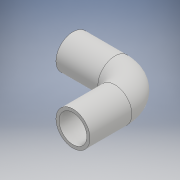
# Autodesk Inventor part: Effector Wire Conduit
Saved by Autodesk Inventor 2018 (Build 220112000, 112)
## iProperties
Created: 2018-05-02
Part Number: Effector Wire Conduit
Material: Generic
Document SubType Name: Modeling
Designer: elect
Density: 1 g/cm^3
Appearance: Default
Author: elect
Autodesk Inventor part; units mm, degrees
ref_plane "YZ Plane" through (0, 0, 0) normal (1, 0, 0) x (0, 1, 0)
ref_plane "XZ Plane" through (0, 0, 0) normal (0, 1, 0) x (-1, 0, 0)
ref_plane "XY Plane" through (0, 0, 0) normal (0, 0, 1) x (1, 0, 0)
sketch "Sketch1" plane through (0, 0, 0) normal (0, 1, 0) x (-1, 0, 0)
  circle A0 centre (0, 0) radius 8.125
  circle A1 centre (0, 0) radius 6.625
  dimension "d0" = 16.25
  dimension "d1" = 13.25
  constraints: 2 centre point, 2 coincident
  measures "d0" diameter of A0
  measures "d1" diameter of A1
sketch "Sketch3" plane through (0, 0, 0) normal (0, 0, 1) x (1, 0, 0)
  line L0 (8.125, 0) -> (8.125, 20)
  line L1 (8.125, 0) -> (28.125, 0) construction
  arc A0 (8.125, 20) -> (-11.875, 40) centre (-11.875, 20) ccw
  line L2 (-11.875, 40) -> (-31.875, 40)
  point P0 (0, 0)
  dimension "d5" = 20
  dimension "d6" = 90
  dimension "d7" = 20
  dimension "d10" = 20
  constraints: 6 end point, 2 horizontal, 2 point on circle, 1 centre point, 1 perpendicular, 1 tangent, 1 vertical
  measures "d5" distance of L0.start L0.end
  measures "d6" angle of L1 L0
  measures "d7" radius of A0
  measures "d10" distance of L2.start L2.end
sweep "Sweep1" add profiles "Sketch1" path "Sketch3"
body "Solid1"
